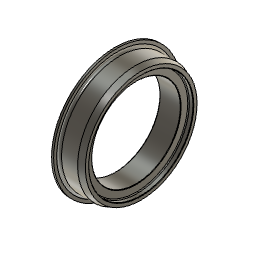
504 v1 (Autodesk Fusion 360 design; units mm, degrees)
Autodesk Fusion 360 part; units mm, degrees
sketch "Sketch1" plane through (0, 0, 0) normal (0, 0, 1) x (1, 0, 0)
  line L0 (20, 60) -> (166.8779, 60) construction
  line L1 (40, 91.5) -> (40.1, 91.5)
  line L2 (20, 91.5) -> (21, 91.5)
  line L3 (21, 91.5) -> (21, 89.95)
  arc A0 (21, 89.95) -> (22.2, 88.75) centre (22.2, 89.95) ccw
  line L4 (22.2, 88.75) -> (30.2, 88.75)
  line L5 (30.2, 88.75) -> (33.0155, 87.7252)
  line L6 (33.0155, 87.7252) -> (33.0187, 86.1004)
  arc A1 (32.8187, 85.9) -> (33.0187, 86.1004) centre (32.8187, 86.1) ccw
  line L7 (32.8191, 85.9) -> (31.0191, 85.8965)
  arc A2 (31.0191, 85.8965) -> (30.6199, 85.4957) centre (31.0199, 85.4965) ccw
  line L8 (20, 91.5) -> (20, 84)
  line L9 (20, 84) -> (19.9, 84)
  line L10 (19.9, 84) -> (19.9, 82.5)
  line L11 (19.9, 82.5) -> (20.4, 82)
  line L12 (20.4, 82) -> (30.4267, 82.0197)
  line L13 (30.6199, 85.4957) -> (30.6263, 82.22)
  line L14 (30.6699, 60) -> (30.6699, 59.9957)
  arc A3 (30.4267, 82.0197) -> (30.6263, 82.22) centre (30.4263, 82.2197) ccw
  dimension "d6" = 31.5
  dimension "d7" = 1
  dimension "d9" = 2.4
  dimension "d10" = 8
  dimension "d11" = 20
  dimension "d15" = 0.4
  dimension "d18" = 0.8
  dimension "d19" = 7.5
  dimension "d20" = 0.1
  dimension "d21" = 1.5
  dimension "d24" = 0.4
  constraint horizontal L0
  constraint horizontal L1
  constraint tangent L3 A0
  constraint tangent A0 L4
  constraint horizontal L4
  constraint tangent L6 A1
  constraint perpendicular L6 L7
  constraint tangent A1 L7
  constraint coincident A1 L7.start
  constraint perpendicular L7 L13
  constraint tangent L7 A2
  constraint tangent A2 L13
  constraint perpendicular L8 L9
  constraint perpendicular L9 L10
  constraint perpendicular L12 L13
  constraint coincident L0 L14.start
  constraint collinear L13 L14
  constraint tangent L13 A3
  constraint tangent L12 A3
  measures "d6" distance of L0.start L2.start
  measures "d7" distance of L2.start L2.end
  measures "d9" diameter of A0
  measures "d10" distance of A0.end L4.end
  measures "d11" angle of L4 L5
  measures "d15" diameter of A1
  measures "d18" diameter of A2
  measures "d19" distance of L2.start L8.end
  measures "d20" distance of L8.end L9.end
  measures "d21" distance of L9.end L10.end
  measures "d24" diameter of A3
revolve "Revolve1" add sketch "Sketch1" angle 360 about axis through (20, 60, 0) along (1, 0, 0)
equation "d6 = ( 63 / 2 ) * 1 mm"
